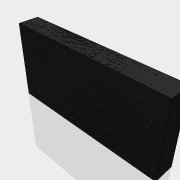
# Autodesk Inventor part: ЛЦМК000002.00.00.00.00.09
Saved by Autodesk Inventor 2021.2 (Build 252289000, 289)
## iProperties
Created: 2025-10-27
Part Number: ЛЦМК000002.00.00.00.00.09
Material: Типовые
Document SubType Name: Modeling
Designer: Захаров
Density: 1 g/cm^3
Appearance: По умолчанию
Author: Захаров
Autodesk Inventor part; units mm, degrees
ref_plane "YZ Plane" through (0, 0, 0) normal (1, 0, 0) x (0, 1, 0)
ref_plane "XZ Plane" through (0, 0, 0) normal (0, 1, 0) x (-1, 0, 0)
ref_plane "XY Plane" through (0, 0, 0) normal (0, 0, 1) x (1, 0, 0)
ref_plane "РабПлоскость1" through (0, 0, -198) normal (0, 0, -1) x (-1, 0, 0)
sketch "Эскиз1" plane through (0, 0, -198) normal (0, 0, -1) x (-1, 0, 0)
  line L0 (-69, 110.895) -> (69, 110.895)
  line L1 (69, 110.895) -> (69, 43.895)
  line L2 (69, 43.895) -> (-69, 43.895)
  line L3 (-69, 43.895) -> (-69, 110.895)
  line L4 (-69, 110.895) -> (69, 43.895) construction
  line L5 (69, 110.895) -> (-69, 43.895) construction
  point P0 (0, 0)
  point P1 (0, 77.395)
  dimension "d0" = 138
  dimension "d1" = 67
  constraints: 12 end point, 2 midpoint, 2 parallel, 1 horizontal, 1 perpendicular
  measures "d0" distance of L1.end L2.end
  measures "d1" distance of L0.end L1.end
extrude "Выдавливание1" add sketch "Эскиз1" along normal blind 18
